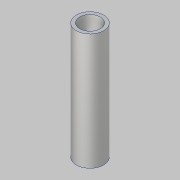
# Autodesk Inventor part: PlaceholderLarge
Saved by Autodesk Inventor 2019.2 (Build 232265000, 265)
## iProperties
Created: 2019-01-12
Part Number: PlaceholderLarge
Material: Aluminium 6061
Document SubType Name: Modeling
Designer: Lion
Density: 2.7 g/cm^3
Appearance: Aluminium - flach
Mass: 0.12363 g
Surface Area: 3.23977 cm^2
Volume: 0.116632 cm^3
Author: Lion
Autodesk Inventor part; units mm, degrees
ref_plane "YZ Plane" through (0, 0, 0) normal (1, 0, 0) x (0, 1, 0)
ref_plane "XZ Plane" through (0, 0, 0) normal (0, 1, 0) x (-1, 0, 0)
ref_plane "XY Plane" through (0, 0, 0) normal (0, 0, 1) x (1, 0, 0)
sketch "Skizze1" plane through (0, 0, 0) normal (0, 1, 0) x (-1, 0, 0)
  circle A0 centre (0, 0) radius 2
  circle A1 centre (0, 0) radius 1.5
  dimension "d5" = 0.5
  dimension "d6" = 4
  constraints: 2 centre point, 2 coincident
  measures "d5" radial gap between concentric circles of A0 A1
  measures "d6" diameter of A0
extrude "Extrusion1" add sketch "Skizze1" along normal blind 17
